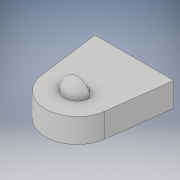
# Autodesk Inventor part: Steitenteil_kabel
Saved by Autodesk Inventor 2019 (Build 230136000, 136)
## iProperties
Created: 2021-12-15
Part Number: Steitenteil_kabel
Material: Generisch
Document SubType Name: Modeling
Designer: Bergi
Density: 1 g/cm^3
Appearance: Vorgabe
Author: Bergi
Autodesk Inventor part; units mm, degrees
note: some values were not read from the file. Chosen so that the rebuilt part matches the saved one: direction of "Bohrung1"; direction of "Bohrung2".
ref_plane "YZ Plane" through (0, 0, 0) normal (1, 0, 0) x (0, 1, 0)
ref_plane "XZ Plane" through (0, 0, 0) normal (0, 1, 0) x (-1, 0, 0)
ref_plane "XY Plane" through (0, 0, 0) normal (0, 0, 1) x (1, 0, 0)
sketch "Skizze1" plane through (0, 0, 0) normal (0, 1, 0) x (-1, 0, 0)
  arc A0 (12.3985, 1.5897) -> (0, 12.5) centre (0, 0) ccw
  line L0 (0, -34.7678) -> (0, 23.1071) construction
  line L1 (12.3985, 1.5897) -> (16, -26.5)
  line L2 (16, -26.5) -> (0, -26.5)
  arc A1 (0, 12.5) -> (-12.3985, 1.5897) centre (0, 0) ccw
  line L3 (-12.3985, 1.5897) -> (-16, -26.5)
  line L4 (-16, -26.5) -> (0, -26.5)
  line L5 (15.4871, -22.5) -> (-15.4871, -22.5)
  dimension "d0" = 25
  dimension "d1" = 32
  dimension "d2" = 39
  dimension "d3" = 35
  constraints: 10 end point, 4 point on circle, 4 point on line, 2 centre point, 2 symmetric about line, 1 coincident, 1 horizontal, 1 perpendicular, 1 tangent, 1 other
  measures "d0" diameter of A0
  measures "d1" distance of L1.end L3.end
  measures "d2" distance from line of L4 A0.end
  measures "d3" distance from line of L5 A0.end
extrude "Extrusion1" add sketch "Skizze1" along normal blind 9.5 contours L1 L5 L3 A1 A0
hole "Bohrung1" at (0, 0, 0) direction (0, 1, 0) diameter 4 depth 9.5
sketch "Skizze2" plane through (0, 9.5, 0) normal (0, 1, 0) x (1, 0, 0)
  line L0 (0, 29.5) -> (0, -19.5) projected
  arc A0 (-5, 0) -> (0, -5) centre (0, 0) ccw
  line L1 (-21.682, 0) -> (21.682, 0) projected
  circle A1 centre (0, 0) radius 2 projected
  line L2 (0, -5) -> (0, -2)
  line L3 (-2, 0) -> (-5, 0)
  point P0 (0, 5)
  dimension "d6" = 10
  constraints: 4 end point, 4 point on circle, 3 point on line, 1 centre point, 1 coincident, 1 collinear, 1 midpoint
  measures "d6" diameter of A0
revolve "Umdrehung1" add sketch "Skizze2" angle 180 about axis through (0, 9.5, 0) along (0, 0, -1) contours L0 A0 L1 A1
fillet "Rundung1" radius 1.5 4 edges at (-1.4142, 9.5, -1.4142) (1.4142, 9.5, -1.4142) (-1.4142, 9.5, 1.4142) (1.4142, 9.5, 1.4142)
sketch "Skizze3" plane through (15.4871, 0, -22.5) normal (0, 0, -1) x (-1, 0, 0)
  line L0 (0, 0) -> (30.9743, 0) projected
  line L1 (30.9743, 0) -> (30.9743, 9.5) projected
  line L2 (0, 9.5) -> (30.9743, 9.5) projected
  line L3 (0, 0) -> (0, 9.5) projected
  line L4 (3.0886, 9.5) -> (0, 9.5) projected
  line L5 (0, 9.5) -> (30.9743, 0) construction
  line L6 (30.9743, 9.5) -> (0, 0) construction
  point P0 (15.4871, 0)
  point P1 (15.4871, 4.75)
  constraints: 4 end point, 1 midpoint
hole "Bohrung2" at (0, 4.75, -22.5) direction (0, 0, 1) diameter 3 end up to surface counterbore diameter 6 counterbore depth 7
